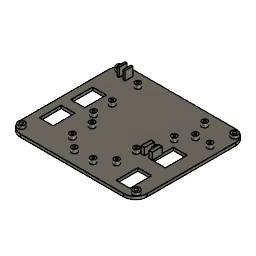
Module base (Autodesk Fusion 360 design; units mm, degrees)
part number: 2026-06-25-19-25-22-878
Autodesk Fusion 360 part; units mm, degrees
sketch "Sketch1" plane through (0, 0, 0) normal (0, 0, 1) x (1, 0, 0)
  line L0 (64.5, 57) -> (-64.5, 57)
  line L1 (-64.5, 57) -> (-64.5, -57)
  line L2 (-64.5, -57) -> (64.5, -57)
  line L3 (64.5, -57) -> (64.5, 57)
extrude "Extrude1" add sketch "Sketch1" along normal blind 3
fillet "Fillet1" radius 12 4 edges at (64.5, -57, 1.5) (-64.5, -57, 1.5) (-64.5, 57, 1.5) (64.5, 57, 1.5)
sketch "Sketch2" plane through (0, 0, 0) normal (0, 0, 1) x (1, 0, 0)
  line L0 (-43, 21) -> (-57, 21)
  line L1 (-57, 21) -> (-57, -1)
  line L2 (-57, -1) -> (-43, -1)
  line L3 (-43, -1) -> (-43, 21)
extrude "Extrude2" cut sketch "Sketch2" along normal blind 5 from surface at -1
sketch "Sketch3" plane through (0, 0, 0) normal (0, 0, 1) x (1, 0, 0)
  line L0 (-43, -11) -> (-57, -11)
  line L1 (-57, -11) -> (-57, -33)
  line L2 (-57, -33) -> (-43, -33)
  line L3 (-43, -33) -> (-43, -11)
extrude "Extrude3" cut sketch "Sketch3" along normal blind 5 from surface at -1
sketch "Sketch4" plane through (0, 0, 0) normal (0, 0, 1) x (1, 0, 0)
  line L0 (51, -27) -> (37, -27)
  line L1 (37, -27) -> (37, -49)
  line L2 (37, -49) -> (51, -49)
  line L3 (51, -49) -> (51, -27)
extrude "Extrude4" cut sketch "Sketch4" along normal blind 5 from surface at -1
sketch "Sketch5" plane through (0, 0, 0) normal (0, 0, 1) x (1, 0, 0)
  line L0 (51, 9) -> (37, 9)
  line L1 (37, 9) -> (37, -13)
  line L2 (37, -13) -> (51, -13)
  line L3 (51, -13) -> (51, 9)
extrude "Extrude5" cut sketch "Sketch5" along normal blind 5 from surface at -1
sketch "Sketch6" plane through (0, 0, 0) normal (0, 0, 1) x (1, 0, 0)
  circle A0 centre (-58.5, 50) radius 3.5
extrude "Extrude6" add sketch "Sketch6" along normal blind 3 from surface at 3
sketch "Sketch7" plane through (0, 0, 0) normal (0, 0, 1) x (1, 0, 0)
  circle A0 centre (-58.5, 50) radius 1.7
extrude "Extrude7" cut sketch "Sketch7" along normal blind 8 from surface at -1
sketch "Sketch8" plane through (0, 0, 0) normal (0, 0, 1) x (1, 0, 0)
  circle A0 centre (-58.5, 50) radius 3
extrude "Extrude8" cut sketch "Sketch8" along normal blind 1.5
sketch "Sketch9" plane through (0, 0, 0) normal (0, 0, 1) x (1, 0, 0)
  circle A0 centre (58.5, 50) radius 3.5
extrude "Extrude9" add sketch "Sketch9" along normal blind 3 from surface at 3
sketch "Sketch10" plane through (0, 0, 0) normal (0, 0, 1) x (1, 0, 0)
  circle A0 centre (58.5, 50) radius 1.7
extrude "Extrude10" cut sketch "Sketch10" along normal blind 8 from surface at -1
sketch "Sketch11" plane through (0, 0, 0) normal (0, 0, 1) x (1, 0, 0)
  circle A0 centre (58.5, 50) radius 3
extrude "Extrude11" cut sketch "Sketch11" along normal blind 1.5
sketch "Sketch12" plane through (0, 0, 0) normal (0, 0, 1) x (1, 0, 0)
  circle A0 centre (-58.5, -50) radius 3.5
extrude "Extrude12" add sketch "Sketch12" along normal blind 3 from surface at 3
sketch "Sketch13" plane through (0, 0, 0) normal (0, 0, 1) x (1, 0, 0)
  circle A0 centre (-58.5, -50) radius 1.7
extrude "Extrude13" cut sketch "Sketch13" along normal blind 8 from surface at -1
sketch "Sketch14" plane through (0, 0, 0) normal (0, 0, 1) x (1, 0, 0)
  circle A0 centre (-58.5, -50) radius 3
extrude "Extrude14" cut sketch "Sketch14" along normal blind 1.5
sketch "Sketch15" plane through (0, 0, 0) normal (0, 0, 1) x (1, 0, 0)
  circle A0 centre (58.5, -50) radius 3.5
extrude "Extrude15" add sketch "Sketch15" along normal blind 3 from surface at 3
sketch "Sketch16" plane through (0, 0, 0) normal (0, 0, 1) x (1, 0, 0)
  circle A0 centre (58.5, -50) radius 1.7
extrude "Extrude16" cut sketch "Sketch16" along normal blind 8 from surface at -1
sketch "Sketch17" plane through (0, 0, 0) normal (0, 0, 1) x (1, 0, 0)
  circle A0 centre (58.5, -50) radius 3
extrude "Extrude17" cut sketch "Sketch17" along normal blind 1.5
sketch "Sketch18" plane through (0, 0, 0) normal (0, 0, 1) x (1, 0, 0)
  circle A0 centre (-31.5, -3.5) radius 2.75
extrude "Extrude18" add sketch "Sketch18" along normal blind 4 from surface at 3
sketch "Sketch19" plane through (0, 0, 0) normal (0, 0, 1) x (1, 0, 0)
  circle A0 centre (-31.5, -3.5) radius 1.1
extrude "Extrude19" cut sketch "Sketch19" along normal blind 5 from surface at 3
sketch "Sketch20" plane through (0, 0, 0) normal (0, 0, 1) x (1, 0, 0)
  circle A0 centre (31.5, -3.5) radius 2.75
extrude "Extrude20" add sketch "Sketch20" along normal blind 4 from surface at 3
sketch "Sketch21" plane through (0, 0, 0) normal (0, 0, 1) x (1, 0, 0)
  circle A0 centre (31.5, -3.5) radius 1.1
extrude "Extrude21" cut sketch "Sketch21" along normal blind 5 from surface at 3
sketch "Sketch22" plane through (0, 0, 0) normal (0, 0, 1) x (1, 0, 0)
  circle A0 centre (-31.5, 15.5) radius 2.75
extrude "Extrude22" add sketch "Sketch22" along normal blind 4 from surface at 3
sketch "Sketch23" plane through (0, 0, 0) normal (0, 0, 1) x (1, 0, 0)
  circle A0 centre (-31.5, 15.5) radius 1.1
extrude "Extrude23" cut sketch "Sketch23" along normal blind 5 from surface at 3
sketch "Sketch24" plane through (0, 0, 0) normal (0, 0, 1) x (1, 0, 0)
  circle A0 centre (31.5, 15.5) radius 2.75
extrude "Extrude24" add sketch "Sketch24" along normal blind 4 from surface at 3
sketch "Sketch25" plane through (0, 0, 0) normal (0, 0, 1) x (1, 0, 0)
  circle A0 centre (31.5, 15.5) radius 1.1
extrude "Extrude25" cut sketch "Sketch25" along normal blind 5 from surface at 3
sketch "Sketch26" plane through (0, 0, 0) normal (0, 0, 1) x (1, 0, 0)
  circle A0 centre (-22.5, -34) radius 2.75
extrude "Extrude26" add sketch "Sketch26" along normal blind 4 from surface at 3
sketch "Sketch27" plane through (0, 0, 0) normal (0, 0, 1) x (1, 0, 0)
  circle A0 centre (-22.5, -34) radius 1.1
extrude "Extrude27" cut sketch "Sketch27" along normal blind 5 from surface at 3
sketch "Sketch28" plane through (0, 0, 0) normal (0, 0, 1) x (1, 0, 0)
  circle A0 centre (22.5, -34) radius 2.75
extrude "Extrude28" add sketch "Sketch28" along normal blind 4 from surface at 3
sketch "Sketch29" plane through (0, 0, 0) normal (0, 0, 1) x (1, 0, 0)
  circle A0 centre (22.5, -34) radius 1.1
extrude "Extrude29" cut sketch "Sketch29" along normal blind 5 from surface at 3
sketch "Sketch30" plane through (0, 0, 0) normal (0, 0, 1) x (1, 0, 0)
  circle A0 centre (-22.5, -14) radius 2.75
extrude "Extrude30" add sketch "Sketch30" along normal blind 4 from surface at 3
sketch "Sketch31" plane through (0, 0, 0) normal (0, 0, 1) x (1, 0, 0)
  circle A0 centre (-22.5, -14) radius 1.1
extrude "Extrude31" cut sketch "Sketch31" along normal blind 5 from surface at 3
sketch "Sketch32" plane through (0, 0, 0) normal (0, 0, 1) x (1, 0, 0)
  circle A0 centre (22.5, -14) radius 2.75
extrude "Extrude32" add sketch "Sketch32" along normal blind 4 from surface at 3
sketch "Sketch33" plane through (0, 0, 0) normal (0, 0, 1) x (1, 0, 0)
  circle A0 centre (22.5, -14) radius 1.1
extrude "Extrude33" cut sketch "Sketch33" along normal blind 5 from surface at 3
sketch "Sketch34" plane through (0, 0, 0) normal (0, 0, 1) x (1, 0, 0)
  circle A0 centre (-34, 44) radius 2.75
extrude "Extrude34" add sketch "Sketch34" along normal blind 4 from surface at 3
sketch "Sketch35" plane through (0, 0, 0) normal (0, 0, 1) x (1, 0, 0)
  circle A0 centre (-34, 44) radius 1.1
extrude "Extrude35" cut sketch "Sketch35" along normal blind 5 from surface at 3
sketch "Sketch36" plane through (0, 0, 0) normal (0, 0, 1) x (1, 0, 0)
  circle A0 centre (34, 44) radius 2.75
extrude "Extrude36" add sketch "Sketch36" along normal blind 4 from surface at 3
sketch "Sketch37" plane through (0, 0, 0) normal (0, 0, 1) x (1, 0, 0)
  circle A0 centre (34, 44) radius 1.1
extrude "Extrude37" cut sketch "Sketch37" along normal blind 5 from surface at 3
sketch "Sketch38" plane through (0, 0, 0) normal (0, 0, 1) x (1, 0, 0)
  circle A0 centre (-9.5, -45) radius 2.75
extrude "Extrude38" add sketch "Sketch38" along normal blind 4 from surface at 3
sketch "Sketch39" plane through (0, 0, 0) normal (0, 0, 1) x (1, 0, 0)
  circle A0 centre (-9.5, -45) radius 1.1
extrude "Extrude39" cut sketch "Sketch39" along normal blind 5 from surface at 3
sketch "Sketch40" plane through (0, 0, 0) normal (0, 0, 1) x (1, 0, 0)
  circle A0 centre (9.5, -45) radius 2.75
extrude "Extrude40" add sketch "Sketch40" along normal blind 4 from surface at 3
sketch "Sketch41" plane through (0, 0, 0) normal (0, 0, 1) x (1, 0, 0)
  circle A0 centre (9.5, -45) radius 1.1
extrude "Extrude41" cut sketch "Sketch41" along normal blind 5 from surface at 3
sketch "Sketch42" plane through (0, 0, 0) normal (0, 0, 1) x (1, 0, 0)
  circle A0 centre (40.5, 28) radius 2.75
extrude "Extrude42" add sketch "Sketch42" along normal blind 4 from surface at 3
sketch "Sketch43" plane through (0, 0, 0) normal (0, 0, 1) x (1, 0, 0)
  circle A0 centre (40.5, 28) radius 1.1
extrude "Extrude43" cut sketch "Sketch43" along normal blind 5 from surface at 3
sketch "Sketch44" plane through (0, 0, 0) normal (0, 0, 1) x (1, 0, 0)
  circle A0 centre (55.5, 28) radius 2.75
extrude "Extrude44" add sketch "Sketch44" along normal blind 4 from surface at 3
sketch "Sketch45" plane through (0, 0, 0) normal (0, 0, 1) x (1, 0, 0)
  circle A0 centre (55.5, 28) radius 1.1
extrude "Extrude45" cut sketch "Sketch45" along normal blind 5 from surface at 3
sketch "Sketch46" plane through (0, 0, 0) normal (0, 0, 1) x (1, 0, 0)
  line L0 (-52, 51) -> (-54, 51)
  line L1 (-54, 51) -> (-54, 43)
  line L2 (-54, 43) -> (-52, 43)
  line L3 (-52, 43) -> (-52, 51)
extrude "Extrude46" add sketch "Sketch46" along normal blind 9 from surface at 3
sketch "Sketch47" plane through (0, 0, 0) normal (0, 0, 1) x (1, 0, 0)
  line L0 (-46, 51) -> (-48, 51)
  line L1 (-48, 51) -> (-48, 43)
  line L2 (-48, 43) -> (-46, 43)
  line L3 (-46, 43) -> (-46, 51)
extrude "Extrude47" add sketch "Sketch47" along normal blind 9 from surface at 3
sketch "Sketch48" plane through (0, 0, 0) normal (0, 0, 1) x (1, 0, 0)
  line L0 (29.75, -3) -> (26.25, -3)
  line L1 (26.25, -3) -> (26.25, -13)
  line L2 (26.25, -13) -> (29.75, -13)
  line L3 (29.75, -13) -> (29.75, -3)
extrude "Extrude48" add sketch "Sketch48" along normal blind 7 from surface at 3
sketch "Sketch49" plane through (0, 0, 0) normal (0, 0, 1) x (1, 0, 0)
  line L0 (37.75, -3) -> (34.25, -3)
  line L1 (34.25, -3) -> (34.25, -13)
  line L2 (34.25, -13) -> (37.75, -13)
  line L3 (37.75, -13) -> (37.75, -3)
extrude "Extrude49" add sketch "Sketch49" along normal blind 7 from surface at 3
named bodies: "FIR Bottom Plate"
